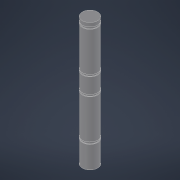
# Autodesk Inventor part: P005-Axe_piston
Saved by Autodesk Inventor 2021.3 (Build 253353000, 353)
## iProperties
Created: 2022-03-30
Part Number: P005-Axe_piston
Material: Aluminium
Document SubType Name: Modeling
Designer: Rémi & Elise
Density: 2.7 g/cm^3
Appearance: Aluminum - Dark
Mass: 0.477129 g
Surface Area: 2.49757 cm^2
Volume: 0.176715 cm^3
Author: Rémi & Elise
Title: Axe piston
Autodesk Inventor part; units mm, degrees
ref_plane "YZ Plane" through (0, 0, 0) normal (1, 0, 0) x (0, 1, 0)
ref_plane "XZ Plane" through (0, 0, 0) normal (0, 1, 0) x (-1, 0, 0)
ref_plane "XY Plane" through (0, 0, 0) normal (0, 0, 1) x (1, 0, 0)
sketch "Sketch2" plane through (0, 0, 0) normal (0, 0, 1) x (1, 0, 0)
  line L0 (-2.1, 0) -> (2.1, 0) construction
  line L1 (0, -2.1) -> (0, 2.1) construction
  circle A0 centre (0, 0) radius 1.5
  dimension "d0" = 3
  constraints: 1 centre point, 1 coincident
  measures "d0" diameter of A0
extrude "Extrusion1" add sketch "Sketch2" along normal blind 25
sketch "Sketch5" plane through (0, 0, 0) normal (0, 1, 0) x (-1, 0, 0)
  line L0 (6.2315, 4.3334) -> (-2.0965, 4.3334) construction
  line L1 (-2.0965, 24.2483) -> (6.2315, 24.2483) construction
  line L2 (1.5, 0) -> (-1.5, 0) construction
  line L3 (1.5, 25) -> (-1.5, 25) construction
  line L4 (1.5, 0) -> (1.5, 25) projected
  line L5 (1.5, 4.3334) -> (1.35, 4.3334)
  line L6 (1.35, 4.3334) -> (1.35, 4.7334)
  line L7 (1.35, 4.7334) -> (1.5, 4.7334)
  line L8 (1.5, 4.7334) -> (1.5, 4.3334)
  line L9 (1.5, 24.2483) -> (1.35, 24.2483)
  line L10 (1.35, 24.2483) -> (1.35, 23.8483)
  line L11 (1.35, 23.8483) -> (1.5, 23.8483)
  line L12 (1.5, 23.8483) -> (1.5, 24.2483)
  line L13 (0, 0) -> (0, 25)
  line L14 (0, 4.3334) -> (0, 14.2908) construction
  line L15 (0, 14.2908) -> (0, 24.2483) construction
  line L16 (0, 14.2908) -> (0, 12.7908) construction
  line L17 (0, 14.2908) -> (0, 15.7908) construction
  line L18 (1.5, 0) -> (1.5, 25) projected
  line L19 (1.5, 12.7908) -> (1.35, 12.7908)
  line L20 (1.35, 12.7908) -> (1.35, 12.3908)
  line L21 (1.35, 12.3908) -> (1.5, 12.3908)
  line L22 (1.5, 12.3908) -> (1.5, 12.7908)
  line L23 (1.5, 0) -> (1.5, 25) projected
  line L24 (1.5, 15.7908) -> (1.35, 15.7908)
  line L25 (1.35, 15.7908) -> (1.35, 16.1908)
  line L26 (1.35, 16.1908) -> (1.5, 16.1908)
  line L27 (1.5, 16.1908) -> (1.5, 15.7908)
  point P0 (1.425, 12.7908)
  point P1 (1.425, 15.7908)
  dimension "d3" = 2.7
  dimension "d4" = 0.4
  dimension "d7" = 3
  constraints: 42 end point, 17 equal length, 9 point on line, 4 horizontal, 4 perpendicular, 3 midpoint, 2 collinear, 2 horizontal alignment, 2 other
  measures "d3" diameter of L6 L13
  measures "d4" distance of L5.end L6.end
  measures "d7" distance of L17.end L16.end
revolve "Revolution1" cut sketch "Sketch5" angle 360 about axis through (0, 0, 0) along (0, 0, 1)
body "Solid1"
